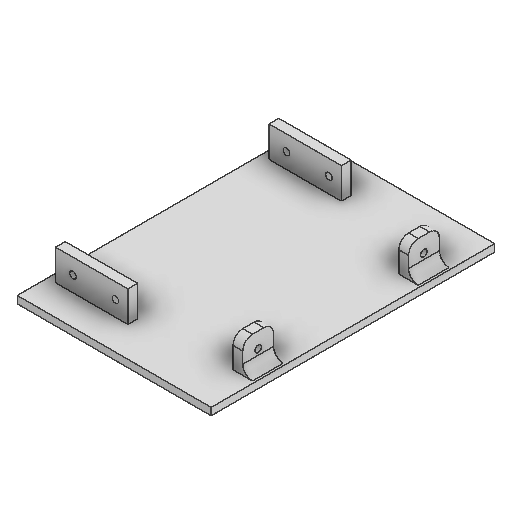
# Autodesk Inventor part: lowerSkidPlate
Saved by Autodesk Inventor 2025 (Build 290162000, 162)
## iProperties
Created: 2025-01-05
Part Number: lowerSkidPlate
Material: Generic
Document SubType Name: Modeling
Designer: derm
Density: 1 g/cm^3
Appearance: Default
Author: derm
Autodesk Inventor part; units mm, degrees
ref_plane "YZ Plane" through (0, 0, 0) normal (1, 0, 0) x (0, 1, 0)
ref_plane "XZ Plane" through (0, 0, 0) normal (0, 1, 0) x (-1, 0, 0)
ref_plane "XY Plane" through (0, 0, 0) normal (0, 0, 1) x (1, 0, 0)
sketch "Sketch1" plane through (0, 0, 0) normal (0, 1, 0) x (-1, 0, 0)
  line L0 (-80, 117) -> (80, 117)
  line L1 (80, 117) -> (80, -117)
  line L2 (80, -117) -> (-80, -117)
  line L3 (-80, -117) -> (-80, 117)
  line L4 (-80, 117) -> (80, -117) construction
  line L5 (80, 117) -> (-80, -117) construction
  point P0 (0, 0)
  dimension "d0" = 160
  dimension "d1" = 234
  constraints: 12 end point, 2 midpoint, 2 parallel, 1 horizontal, 1 perpendicular
  measures "d0" distance of L1.end L2.end
  measures "d1" distance of L0.end L1.end
extrude "Extrusion1" add sketch "Sketch1" along normal blind 6
sketch "Sketch2" plane through (0, 6, 0) normal (0, 1, 0) x (1, 0, 0)
  line L0 (80, 117) -> (-80, 117) projected
  line L1 (-80, 117) -> (-80, -117) projected
  line L2 (-80, -117) -> (80, -117) projected
  line L3 (80, -117) -> (80, 117) projected
  line L4 (76.2612, -82.1) -> (62.1597, -82.1) projected
  line L5 (62.1597, 116.5) -> (62.1597, -117.5) projected
  line L6 (62.1597, -82.1) -> (70.1597, -82.1)
  line L7 (70.1597, -82.1) -> (70.1597, -55.7)
  line L8 (70.1597, -55.7) -> (62.1597, -55.7)
  line L9 (62.1597, -55.7) -> (62.1597, -82.1)
  line L10 (70.1597, -82.1) -> (62.1597, -82.1)
  line L11 (62.1597, -82.1) -> (62.1597, -81.1)
  line L12 (62.1597, -81.1) -> (70.1597, -81.1)
  line L13 (70.1597, -81.1) -> (70.1597, -82.1)
  point P0 (0, 0)
  point P1 (66.1597, -55.7)
  point P2 (66.1597, -82.1)
  point P3 (62.1597, -55.7)
  dimension "d4" = 26.4
  dimension "d5" = 8
  dimension "d8" = 1
  constraints: 16 end point, 4 parallel, 2 horizontal, 2 midpoint, 2 perpendicular, 1 point on line
  measures "d4" distance of point (66.16, -55.7) point (66.16, -82.1)
  measures "d5" distance between parallel lines of L5 L7
  measures "d8" distance between parallel lines of L12 L6
extrude "Extrusion2" add sketch "Sketch2" along normal blind 25.4 contours L5 L8 L7 L12
sketch "Sketch3" plane through (70.1597, 6, 81.1) normal (1, 0, 0) x (0, 0, -1)
  line L0 (25.4, 0) -> (0, 0) projected
  line L1 (25.4, 0) -> (25.4, 25.4) projected
  line L2 (0, 25.4) -> (25.4, 25.4) projected
  line L3 (0, 0) -> (0, 25.4) projected
  circle A0 centre (12.7, 12.7) radius 2.75
  point P0 (81.1, -6)
  dimension "d9" = 5.5
  constraints: 1 centre point
  measures "d9" diameter of A0
extrude "Extrusion3" cut sketch "Sketch3" against normal blind 25.4 contours A0
fillet "Fillet1" radius 8 3 edges at (70.1597, 6, 68.4) (66.1597, 31.4, 55.7) (66.1597, 31.4, 81.1)
sketch "Sketch4" plane through (0, 6, 0) normal (0, 1, 0) x (1, 0, 0)
  line L0 (78.1597, -81.1) -> (62.1597, -81.1) projected
  line L1 (62.1597, -81.1) -> (62.1597, -55.7) projected
  line L2 (62.1597, -55.7) -> (78.1597, -55.7) projected
  line L3 (78.1597, -81.1) -> (78.1597, -55.7) projected
  line L4 (80, 117) -> (-80, 117) projected
  line L5 (-80, 117) -> (-80, -117) projected
  line L6 (-80, -117) -> (80, -117) projected
  line L7 (80, -117) -> (80, 117) projected
  line L8 (-217.2403, -92.1) -> (36.7597, -92.1) projected
  line L9 (-7.3833, -87.6172) -> (32.2769, -47.957) projected
  line L10 (-13.6234, -92.1) -> (-73.3252, -92.1)
  line L11 (-73.3252, -92.1) -> (-73.3252, -84.1)
  line L12 (-73.3252, -84.1) -> (-13.6234, -84.1)
  line L13 (-13.6234, -84.1) -> (-13.6234, -92.1)
  point P0 (0, 0)
  point P1 (-73.3252, -92.1)
  dimension "d14" = 8
  constraints: 8 end point, 2 parallel, 1 horizontal, 1 perpendicular, 1 point on line, 1 vertical
  measures "d14" distance between parallel lines of L8 L12
extrude "Extrusion4" add sketch "Sketch4" along normal blind 25.4 contours L11 L12 L13 L8
sketch "Sketch5" plane through (-80, 6, 84.1) normal (0, 0, -1) x (-1, 0, 0)
  line L0 (-6.6748, 0) -> (-66.3766, 0) projected
  line L1 (-6.6748, 0) -> (-6.6748, 25.4) projected
  line L2 (-66.3766, 25.4) -> (-6.6748, 25.4) projected
  line L3 (-66.3766, 0) -> (-66.3766, 25.4) projected
  circle A0 centre (-56.0684, 12.7) radius 2.75
  circle A1 centre (-21.0684, 12.7) radius 2.75
  circle A2 centre (13.9316, 12.7) radius 2.75
  point P0 (-80, -6)
  dimension "d17" = 5.5
  dimension "d22" = 35
  constraints: 3 centre point, 1 horizontal, 4 other
  measures "d17" diameter of A0
  measures "d22" distance of A0.centre A1.centre
extrude "Extrusion5" cut sketch "Sketch5" against normal blind 25.4 contours A0 | A1 | A2
mirror "Mirror1" about plane through (0, 0, 0) normal (0, 0, 1) of "Extrusion2", "Extrusion3", "Fillet1", "Extrusion4", "Extrusion5"
sketch "Sketch6" plane through (0, 6, 0) normal (0, 1, 0) x (1, 0, 0)
  line L0 (-13.6234, 84.1) -> (-73.3252, 84.1) projected
  line L1 (-73.3252, 84.1) -> (-73.3252, 92.1) projected
  line L2 (-73.3252, 92.1) -> (-13.6234, 92.1) projected
  line L3 (-13.6234, 92.1) -> (-13.6234, 84.1) projected
  line L4 (78.1597, 55.7) -> (62.1597, 55.7) projected
  line L5 (62.1597, 55.7) -> (62.1597, 81.1) projected
  line L6 (62.1597, 81.1) -> (78.1597, 81.1) projected
  line L7 (78.1597, 55.7) -> (78.1597, 81.1) projected
  line L8 (-73.3252, -84.1) -> (-13.6234, -84.1) projected
  line L9 (-13.6234, -84.1) -> (-13.6234, -92.1) projected
  line L10 (-13.6234, -92.1) -> (-73.3252, -92.1) projected
  line L11 (-73.3252, -92.1) -> (-73.3252, -84.1) projected
  line L12 (78.1597, -81.1) -> (62.1597, -81.1) projected
  line L13 (62.1597, -81.1) -> (62.1597, -55.7) projected
  line L14 (62.1597, -55.7) -> (78.1597, -55.7) projected
  line L15 (78.1597, -81.1) -> (78.1597, -55.7) projected
  line L16 (80, 117) -> (-80, 117) projected
  line L17 (-80, 117) -> (-80, -117) projected
  line L18 (-80, -117) -> (80, -117) projected
  line L19 (80, -117) -> (80, 117) projected
  line L20 (-14.0403, 77.5) -> (-69.0403, 77.5)
  line L21 (-69.0403, 77.5) -> (-69.0403, -77.5)
  line L22 (-69.0403, -77.5) -> (-14.0403, -77.5)
  line L23 (-14.0403, -77.5) -> (-14.0403, 77.5)
  line L24 (-14.0403, 77.5) -> (-69.0403, -77.5) construction
  line L25 (-69.0403, 77.5) -> (-14.0403, -77.5) construction
  line L26 (80, -117) -> (80, 117) projected
  line L27 (80, 0) -> (-80, 0)
  line L28 (-9.0403, -82.5) -> (-74.0403, -82.5)
  line L29 (-74.0403, -82.5) -> (-74.0403, 82.5)
  line L30 (-74.0403, 82.5) -> (-9.0403, 82.5)
  line L31 (-9.0403, 82.5) -> (-9.0403, -82.5)
  point P0 (0, 0)
  point P1 (-41.5403, 0)
  dimension "d27" = 155
  dimension "d28" = 55
  dimension "d29" = 76.2
  dimension "d30" = 5
  constraints: 22 end point, 4 midpoint, 4 parallel, 2 perpendicular, 1 horizontal, 1 point on line, 3 other
  measures "d27" distance of L22.end L20.start
  measures "d28" distance of L21.end L22.end
  measures "d29" distance between parallel lines of L5 L23
  measures "d30" distance between parallel lines of L31 L23
sketch "Sketch7" plane through (0, 6, 0) normal (0, 1, 0) x (1, 0, 0)
  line L0 (-14.0403, 77.5) -> (-69.0403, 77.5) projected
  line L1 (-69.0403, 77.5) -> (-69.0403, -77.5) projected
  line L2 (-69.0403, -77.5) -> (-14.0403, -77.5) projected
  line L3 (-14.0403, -77.5) -> (-14.0403, 77.5) projected
  point P0 (0, 0)
body "Solid1"
